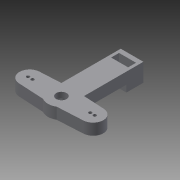
# Autodesk Inventor part: HornPocket
Saved by Autodesk Inventor 2014 SP1 (Build 180222100, 222)
## iProperties
Created: 2017-05-20
Part Number: HornPocket
Material: Generic
Document SubType Name: Modeling
Designer: danielsikar
Density: 1 g/cm^3
Appearance: Default
Author: danielsikar
Autodesk Inventor part; units mm, degrees
ref_plane "YZ Plane" through (0, 0, 0) normal (1, 0, 0) x (0, 1, 0)
ref_plane "Work Plane1" through (-16.55, 6.25, 30.8) normal (0, 0, 1) x (-1, 0, 0)
sketch "Sketch1" plane through (-16.55, 6.25, 30.8) normal (0, 0, 1) x (-1, 0, 0)
  circle A0 centre (4.7413, 0) radius 0.35 projected
  circle A1 centre (6.7413, 0) radius 0.35 projected
  circle A2 centre (8.7413, 0) radius 0.35 projected
  circle A3 centre (10.7413, 0) radius 0.35 projected
  circle A4 centre (12.7413, 0) radius 0.35 projected
  circle A5 centre (14.7413, 0) radius 0.35 projected
  circle A6 centre (-4.7413, 0) radius 0.35 projected
  circle A7 centre (-6.7413, 0) radius 0.35 projected
  circle A8 centre (-8.7413, 0) radius 0.35 projected
  circle A9 centre (-10.7413, 0) radius 0.35 projected
  circle A10 centre (-12.7413, 0) radius 0.35 projected
  circle A11 centre (-14.7413, 0) radius 0.35 projected
  circle A12 centre (0, 0) radius 2.3 projected
  line L0 (2.2091, 2.65) -> (14.1096, 1.997) projected
  arc A13 (2.2091, 2.65) -> (-2.2091, 2.65) centre (0, 0) ccw projected
  line L1 (-14.1096, 1.997) -> (-2.2091, 2.65) projected
  arc A14 (-14.1096, 1.997) -> (-14.1096, -1.997) centre (-14, 0) ccw projected
  line L2 (-2.2091, -2.65) -> (-14.1096, -1.997) projected
  arc A15 (-2.2091, -2.65) -> (2.2091, -2.65) centre (0, 0) ccw projected
  line L3 (14.1096, -1.997) -> (2.2091, -2.65) projected
  arc A16 (14.1096, -1.997) -> (14.1096, 1.997) centre (14, 0) ccw projected
  arc A17 (2.2852, 2.8461) -> (-2.2852, 2.8461) centre (0, 0) ccw
  line L4 (2.2852, 2.8461) -> (14.1205, 2.1967)
  arc A18 (14.1205, -2.1967) -> (14.1205, 2.1967) centre (14, 0) ccw
  line L5 (14.1205, -2.1967) -> (2.2852, -2.8461)
  arc A19 (-2.2852, -2.8461) -> (2.2852, -2.8461) centre (0, 0) ccw
  line L6 (-2.2852, -2.8461) -> (-14.1205, -2.1967)
  arc A20 (-14.1205, 2.1967) -> (-14.1205, -2.1967) centre (-14, 0) ccw
  line L7 (-14.1205, 2.1967) -> (-2.2852, 2.8461)
  arc A21 (3.0522, 5.1075) -> (-3.0522, 5.1075) centre (0, 0) ccw
  line L8 (3.0522, 5.1075) -> (14.2466, 4.4932)
  arc A22 (14.2466, -4.4932) -> (14.2466, 4.4932) centre (14, 0) ccw
  line L9 (14.2466, -4.4932) -> (3.0522, -5.1075)
  arc A23 (-3.0522, -5.1075) -> (3.0522, -5.1075) centre (0, 0) ccw
  line L10 (-3.0522, -5.1075) -> (-14.2466, -4.4932)
  arc A24 (-14.2466, 4.4932) -> (-14.2466, -4.4932) centre (-14, 0) ccw
  line L11 (-14.2466, 4.4932) -> (-3.0522, 5.1075)
  circle A25 centre (-14.7413, 0) radius 0.35 projected
  point P0 (-16.55, 6.25)
  dimension "d0" = 0.2
  dimension "d1" = 2.5
  constraints: 16 end point, 16 point on circle, 8 centre point, 14 other
  measures "d0" distance between parallel lines of L1 L7
  measures "d1" distance between parallel lines of L1 L11
extrude "Extrusion1" add sketch "Sketch1" against normal blind 2.5 contours L8 A22 L9 A23 L10 A24 L11 A21
sketch "Sketch2" plane through (-16.55, 6.25, 30.8) normal (0, 0, 1) x (1, 0, 0)
  arc A0 (-3.0522, -5.1075) -> (3.0522, -5.1075) centre (0, 0) ccw projected
  line L0 (14.2466, -4.4932) -> (3.0522, -5.1075) projected
  arc A1 (14.2466, -4.4932) -> (14.2466, 4.4932) centre (14, 0) ccw projected
  line L1 (3.0522, 5.1075) -> (14.2466, 4.4932) projected
  arc A2 (3.0522, 5.1075) -> (-3.0522, 5.1075) centre (0, 0) ccw projected
  line L2 (-14.2466, 4.4932) -> (-3.0522, 5.1075) projected
  arc A3 (-14.2466, 4.4932) -> (-14.2466, -4.4932) centre (-14, 0) ccw projected
  line L3 (-3.0522, -5.1075) -> (-14.2466, -4.4932) projected
  line L4 (14.1205, -2.1967) -> (2.2852, -2.8461) projected
  arc A4 (-2.2852, -2.8461) -> (2.2852, -2.8461) centre (0, 0) ccw projected
  line L5 (-2.2852, -2.8461) -> (-14.1205, -2.1967) projected
  arc A5 (-14.1205, 2.1967) -> (-14.1205, -2.1967) centre (-14, 0) ccw projected
  line L6 (-14.1205, 2.1967) -> (-2.2852, 2.8461) projected
  arc A6 (2.2852, 2.8461) -> (-2.2852, 2.8461) centre (0, 0) ccw projected
  line L7 (2.2852, 2.8461) -> (14.1205, 2.1967) projected
  arc A7 (14.1205, -2.1967) -> (14.1205, 2.1967) centre (14, 0) ccw projected
  arc A8 (-3.0522, -5.1075) -> (3.0522, -5.1075) centre (0, 0) ccw projected
  line L8 (14.2466, -4.4932) -> (3.0522, -5.1075) projected
  arc A9 (14.2466, -4.4932) -> (14.2466, 4.4932) centre (14, 0) ccw projected
  line L9 (3.0522, 5.1075) -> (14.2466, 4.4932) projected
  arc A10 (3.0522, 5.1075) -> (-3.0522, 5.1075) centre (0, 0) ccw projected
  line L10 (-14.2466, 4.4932) -> (-3.0522, 5.1075) projected
  arc A11 (-14.2466, 4.4932) -> (-14.2466, -4.4932) centre (-14, 0) ccw projected
  line L11 (-3.0522, -5.1075) -> (-14.2466, -4.4932) projected
  circle A12 centre (-14.7413, 0) radius 0.35 projected
  circle A13 centre (-12.7413, 0) radius 0.35 projected
  circle A14 centre (12.7413, 0) radius 0.35 projected
  circle A15 centre (14.7413, 0) radius 0.35 projected
  circle A16 centre (0, 0) radius 2.3 projected
  point P0 (16.55, -6.25)
extrude "Extrusion2" add sketch "Sketch2" along normal blind 2.5 contours L3 A3 L2 A2 L1 A1 L0 A0 | L4 A4 L5 A5 L6 A6 L7 A7
sketch "Sketch3" plane through (-16.55, 6.25, 33.3) normal (0, 0, 1) x (1, 0, 0)
  circle A0 centre (14.7413, 0) radius 0.35 projected
  circle A1 centre (12.7413, 0) radius 0.35 projected
  circle A2 centre (-12.7413, 0) radius 0.35 projected
  circle A3 centre (-14.7413, 0) radius 0.35 projected
  circle A4 centre (-14.7413, 0) radius 0.7
  circle A5 centre (-12.7413, 0) radius 0.7
  circle A6 centre (12.7413, 0) radius 0.7
  circle A7 centre (14.7413, 0) radius 0.7
  point P0 (16.55, -6.25)
  dimension "d6" = 1.4
  dimension "d7" = 1.4
  dimension "d8" = 1.4
  dimension "d9" = 1.4
  constraints: 4 centre point, 4 coincident
  measures "d6" diameter of A4
  measures "d7" diameter of A5
  measures "d8" diameter of A6
  measures "d9" diameter of A7
extrude "Extrusion3" cut sketch "Sketch3" against normal up to next
ref_plane "Work Plane2" through (0, 14.75, 0) normal (0, 1, 0) x (-1, 0, 0)
sketch "Sketch4" plane through (0, 14.75, 0) normal (0, 1, 0) x (-1, 0, 0)
  line L0 (19.6022, 33.3) -> (30.7966, 33.3) construction
  line L1 (30.7966, 28.3) -> (19.6022, 28.3) construction
  line L2 (2.3034, 33.3) -> (13.4978, 33.3) construction
  line L3 (13.4978, 28.3) -> (2.3034, 28.3) construction
  line L4 (11.55, 33.3) -> (21.55, 33.3)
  line L5 (21.55, 33.3) -> (21.55, 28.3)
  line L6 (21.55, 28.3) -> (11.55, 28.3)
  line L7 (11.55, 28.3) -> (11.55, 33.3)
  line L8 (-1.95, 33.3) -> (-1.95, 28.3) construction
  line L9 (35.05, 33.3) -> (35.05, 28.3) construction
  point P0 (0, 0)
  dimension "d13" = 10
  dimension "d14" = 13.5
  constraints: 8 end point, 2 parallel, 2 point on line, 1 horizontal, 1 perpendicular
  measures "d13" distance of L5.end L6.end
  measures "d14" distance between parallel lines of L7 L8
extrude "Extrusion4" add sketch "Sketch4" against normal up to next
sketch "Sketch5" plane through (0, 14.75, 0) normal (0, 1, 0) x (1, 0, 0)
  line L0 (-11.55, -33.3) -> (-21.55, -33.3) projected
  line L1 (-11.55, -28.3) -> (-11.55, -33.3) projected
  line L2 (-21.55, -28.3) -> (-11.55, -28.3) projected
  line L3 (-21.55, -33.3) -> (-21.55, -28.3) projected
  point P0 (0, 0)
extrude "Extrusion5" add sketch "Sketch5" along normal blind 22.7
sketch "Sketch6" plane through (-16.55, 6.25, 28.3) normal (0, 0, -1) x (-1, 0, 0)
  line L0 (-5, 31.2) -> (5, 31.2) projected
  line L1 (-5, 31.2) -> (-5, 5.0006) projected
  line L2 (-3.75, 29.2) -> (3.75, 29.2)
  line L3 (3.75, 29.2) -> (3.75, 25.7)
  line L4 (3.75, 25.7) -> (-3.75, 25.7)
  line L5 (-3.75, 25.7) -> (-3.75, 29.2)
  point P0 (-16.55, -6.25)
  dimension "d19" = 7.5
  dimension "d20" = 3.5
  dimension "d21" = 1.25
  dimension "d22" = 2
  constraints: 8 end point, 2 parallel, 1 horizontal, 1 perpendicular
  measures "d19" distance of L3.end L4.end
  measures "d20" distance of L2.end L3.end
  measures "d21" distance between parallel lines of L5 L1
  measures "d22" distance between parallel lines of L2 L0
extrude "Extrusion6" cut sketch "Sketch6" against normal up to next
sketch "Sketch7" plane through (-16.55, 6.25, 28.3) normal (0, 0, -1) x (-1, 0, 0)
  line L0 (-3.75, 25.7) -> (-3.75, 29.2) projected
  line L1 (-3.75, 29.2) -> (3.75, 29.2) projected
  line L2 (3.75, 29.2) -> (3.75, 25.7) projected
  line L3 (3.75, 25.7) -> (-3.75, 25.7) projected
  line L4 (5, 31.2) -> (5, 5.0006) projected
  line L5 (-5, 31.2) -> (5, 31.2)
  line L6 (5, 31.2) -> (5, 23.7)
  line L7 (5, 23.7) -> (-5, 23.7)
  line L8 (-5, 23.7) -> (-5, 31.2)
  point P0 (-16.55, -6.25)
  dimension "d25" = 7.5
  constraints: 8 end point, 2 parallel, 1 horizontal, 1 perpendicular, 1 point on line
  measures "d25" distance of L5.end L6.end
extrude "Extrusion7" add sketch "Sketch7" along normal blind 3
sketch "Sketch8" plane through (0, 37.45, 0) normal (0, 1, 0) x (1, 0, 0)
  circle A0 centre (-16.55, -29.3) radius 2.15
  point P0 (0, 0)
  dimension "d28" = 4.3
  constraints: 1 centre point
  measures "d28" diameter of A0
extrude "Extrusion8" cut sketch "Sketch8" against normal blind 11
body "Solid1"
